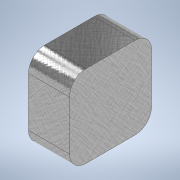
# Autodesk Inventor part: Buttons
Saved by Autodesk Inventor 2022.2 (Build 262287000, 287)
## iProperties
Created: 2022-02-23
Part Number: Buttons
Material: Generic
Document SubType Name: Modeling
Designer: PRASHANTH
Density: 1 g/cm^3
Appearance: Galvanized
Author: PRASHANTH
Autodesk Inventor part; units mm, degrees
ref_plane "YZ Plane" through (0, 0, 0) normal (1, 0, 0) x (0, 1, 0)
ref_plane "XZ Plane" through (0, 0, 0) normal (0, 1, 0) x (-1, 0, 0)
ref_plane "XY Plane" through (0, 0, 0) normal (0, 0, 1) x (1, 0, 0)
sketch "Sketch1" plane through (0, 0, 0) normal (1, 0, 0) x (0, 1, 0)
  line L0 (-3, 5) -> (3, 5)
  line L1 (5, 3) -> (5, -3)
  line L2 (3, -5) -> (-3, -5)
  line L3 (-5, -3) -> (-5, 3)
  line L4 (-5, 5) -> (5, -5) construction
  line L5 (5, 5) -> (-5, -5) construction
  arc A0 (5, 3) -> (3, 5) centre (3, 3) ccw
  arc A1 (3, -5) -> (5, -3) centre (3, -3) ccw
  arc A2 (-3, 5) -> (-5, 3) centre (-3, 3) ccw
  arc A3 (-5, -3) -> (-3, -5) centre (-3, -3) ccw
  point P0 (0, 0)
  dimension "d0" = 10
  dimension "d1" = 10
  dimension "d2" = 2
  dimension "d3" = 2
  constraints: 12 end point, 8 point on circle, 8 point on line, 8 tangent, 4 centre point, 2 equal radius, 2 midpoint, 2 parallel, 1 horizontal, 1 perpendicular
  measures "d0" distance of L4.end L5.end
  measures "d1" distance of L5.start L4.end
  measures "d2" radius of A0
  measures "d3" radius of A1
extrude "Extrusion1" add sketch "Sketch1" along normal blind 5
body "Solid1"
